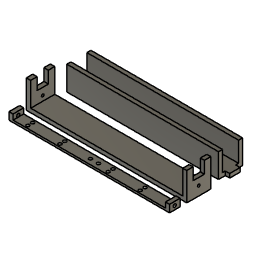
sampApp 20 v19 (Autodesk Fusion 360 design; units mm, degrees)
Autodesk Fusion 360 part; units mm, degrees
note: some values were not read from the file. Chosen so that the rebuilt part matches the saved one: which face or edge a step refers to.
sketch "Sketch1" plane through (0, 0, 0) normal (0, 0, 1) x (1, 0, 0)
  line L0 (0, 0) -> (70, 0)
  line L1 (70, 0) -> (70, 50)
  line L2 (70, 50) -> (0, 50)
  line L3 (0, 50) -> (0, 0)
  constraint horizontal L0
  constraint vertical L1
  constraint horizontal L2
  constraint vertical L3
  constraint coincident L0.start L3.end
extrude "Extrude1" add sketch "Sketch1" along normal blind 5 makes body 1
sketch "Sketch2" plane through (0, 0, 5) normal (0, 0, 1) x (-1, 0, 0)
  line L0 (0, -50) -> (0, 0)
  line L1 (0, 0) -> (-70, 0)
  line L2 (-70, 0) -> (-70, -50)
  line L3 (-70, -50) -> (0, -50)
  line L4 (-65, 0) -> (-70, 0)
  line L5 (-70, 0) -> (-70, -50)
  line L6 (-70, -50) -> (-65, -50)
  line L7 (-65, -50) -> (-65, 0)
  line L8 (0, 0) -> (-5, 0)
  line L9 (-5, 0) -> (-5, -50)
  line L10 (-5, -50) -> (0, -50)
  line L11 (0, -50) -> (0, 0)
  constraint horizontal L4
  constraint vertical L5
  constraint horizontal L6
  constraint vertical L7
  constraint coincident L2.end L3.start
  constraint coincident L1 L4.start
  constraint horizontal L8
  constraint vertical L9
  constraint horizontal L10
  constraint vertical L11
  constraint coincident L3 L9.end
  constraint coincident L0.end L1.start
extrude "Extrude2" add sketch "Sketch2" along normal blind 30 contours L0 L1 L3 L8 L9 L10 L11 | L1 L2 L3 L4 L5 L6 L7 bodies 1
extrude "Extrude3" cut 1 faces at (45, 50, 1.6667) along direction (0, -1, 0) blind 10 on bodies 1 bodies 1
sketch "Sketch3" plane through (0, 0, 0) normal (0, 0, 1) x (1, 0, 0)
  line L0 (5, 45) -> (65, 45)
  line L1 (65, 45) -> (65, 85)
  line L2 (65, 85) -> (5, 85)
  line L3 (5, 85) -> (5, 45)
  constraint horizontal L0
  constraint vertical L1
  constraint horizontal L2
  constraint vertical L3
extrude "Extrude4" add sketch "Sketch3" along normal blind 5 separate body makes body 2
sketch "Sketch4" plane through (0, 0, 5) normal (0, 0, 1) x (-1, 0, 0)
  line L0 (-5, -85) -> (-5, -45)
  line L1 (-5, -45) -> (-65, -45)
  line L2 (-65, -45) -> (-65, -85)
  line L3 (-65, -85) -> (-5, -85)
  line L4 (-65, -45) -> (-5, -45)
  line L5 (-5, -45) -> (-5, -50)
  line L6 (-5, -50) -> (-65, -50)
  line L7 (-65, -50) -> (-65, -45)
  line L8 (-5, -80) -> (-65, -80)
  line L9 (-65, -80) -> (-65, -85)
  line L10 (-65, -85) -> (-5, -85)
  line L11 (-5, -85) -> (-5, -80)
  constraint horizontal L4
  constraint vertical L5
  constraint horizontal L6
  constraint vertical L7
  constraint coincident L0 L5.end
  constraint coincident L1.end L2.start
  constraint horizontal L8
  constraint vertical L9
  constraint horizontal L10
  constraint vertical L11
  constraint coincident L2.end L3.start
  constraint coincident L0 L8.start
extrude "Extrude5" add sketch "Sketch4" along normal blind 25 contours L0 L2 L3 L8 L9 L10 L11 | L0 L1 L2 L4 L5 L6 L7 bodies 2
extrude "Extrude6" cut 1 faces at (5, 70, 1.6667) along direction (1, 0, 0) blind 0.5 on bodies 2 bodies 2
extrude "Extrude7" cut 1 faces at (65, 60, 1.6667) along direction (-1, 0, 0) blind 0.5 on bodies 2 bodies 2
sketch "Sketch5" plane through (0, 0, 35) normal (0, 0, 1) x (-1, 0, 0)
  line L0 (-5, -40) -> (0, -40)
  line L1 (0, -40) -> (0, 0)
  line L2 (0, 0) -> (-5, 0)
  line L3 (-5, 0) -> (-5, -40)
  line L4 (0, -15) -> (-5, -15)
  line L5 (-5, -15) -> (-5, -25)
  line L6 (-5, -25) -> (0, -25)
  line L7 (0, -25) -> (0, -15)
  line L8 (-70, -15) -> (-65, -15)
  line L9 (-65, -15) -> (-65, -25)
  line L10 (-65, -25) -> (-70, -25)
  line L11 (-70, -25) -> (-70, -15)
  constraint horizontal L4
  constraint vertical L5
  constraint horizontal L6
  constraint vertical L7
  constraint coincident L3 L5.end
  constraint coincident L1 L4.start
  constraint horizontal L8
  constraint vertical L9
  constraint horizontal L10
  constraint vertical L11
extrude "Extrude8" cut sketch "Sketch5" against normal blind 10 contours L8 L9 L10 L11 bodies 1
sketch "Sketch6" plane through (0, 0, 35) normal (0, 0, 1) x (-1, 0, 0)
  line L0 (-5, -40) -> (0, -40)
  line L1 (0, -40) -> (0, 0)
  line L2 (0, 0) -> (-5, 0)
  line L3 (-5, 0) -> (-5, -40)
  line L4 (0, -15) -> (-5, -15)
  line L5 (-5, -15) -> (-5, -25)
  line L6 (-5, -25) -> (0, -25)
  line L7 (0, -25) -> (0, -15)
  constraint horizontal L4
  constraint vertical L5
  constraint horizontal L6
  constraint vertical L7
  constraint coincident L3 L5.end
  constraint coincident L1 L4.start
extrude "Extrude9" cut sketch "Sketch6" against normal blind 10 contours L1 L3 L4 L5 L6 L7 bodies 1
sketch "Sketch7" plane through (0, 0, 5) normal (0, 0, 1) x (-1, 0, 0)
  line L0 (-65, -40) -> (-5, -40)
  line L1 (-5, -40) -> (-5, 0)
  line L2 (-5, 0) -> (-65, 0)
  line L3 (-65, 0) -> (-65, -40)
  line L4 (0, 15) -> (-70, 15)
  line L5 (-70, 15) -> (-70, 25)
  line L6 (-70, 25) -> (0, 25)
  line L7 (0, 25) -> (0, 15)
  constraint horizontal L4
  constraint vertical L5
  constraint horizontal L6
  constraint vertical L7
extrude "Extrude10" add sketch "Sketch7" along normal blind 5 separate body contours L4 L5 L6 L7 makes body 3
sketch "Sketch8" plane through (64.5, 0, 0) normal (1, 0, 0) x (0, 1, 0)
  line L0 (45, 0) -> (85, 0)
  line L1 (85, 0) -> (85, 30)
  line L2 (85, 30) -> (80, 30)
  line L3 (80, 30) -> (80, 5)
  line L4 (80, 5) -> (50, 5)
  line L5 (50, 5) -> (50, 30)
  line L6 (50, 30) -> (45, 30)
  line L7 (45, 30) -> (45, 0)
  line L8 (70, 5) -> (60, 5)
  line L9 (60, 5) -> (60, 0)
  line L10 (60, 0) -> (70, 0)
  line L11 (70, 0) -> (70, 5)
  constraint horizontal L8
  constraint vertical L9
  constraint horizontal L10
  constraint vertical L11
  constraint coincident L0 L9.end
  constraint coincident L4 L8.start
extrude "Extrude11" add sketch "Sketch8" along normal blind 7.5 contours L0 L4 L8 L9 L10 L11 bodies 2
extrude "Extrude12" cut 1 faces at (72, 63.3333, 3.3333) along direction (-1, 0, 0) blind 2 on bodies 2 bodies 2
sketch "Sketch9" plane through (5.5, 0, 0) normal (-1, 0, 0) x (0, -1, 0)
  line L0 (-85, 0) -> (-45, 0)
  line L1 (-45, 0) -> (-45, 30)
  line L2 (-45, 30) -> (-50, 30)
  line L3 (-50, 30) -> (-50, 5)
  line L4 (-50, 5) -> (-80, 5)
  line L5 (-80, 5) -> (-80, 30)
  line L6 (-80, 30) -> (-85, 30)
  line L7 (-85, 30) -> (-85, 0)
  line L8 (-60.2501, 5) -> (-70, 5)
  line L9 (-70, 5) -> (-70, 0)
  line L10 (-70, 0) -> (-60.2501, 0)
  line L11 (-60.2501, 0) -> (-60.2501, 5)
  constraint horizontal L8
  constraint vertical L9
  constraint horizontal L10
  constraint vertical L11
  constraint coincident L0 L9.end
  constraint coincident L4 L8.start
extrude "Extrude13" add sketch "Sketch9" along normal blind 5.5 contours L0 L4 L8 L9 L10 L11 bodies 2
move_body "Move1" bodies 3 to x (1, 0, 0) y (0, 1, 0) z (0, 0, 1) at (0, 0, -5)
extrude "Extrude14" cut 2 faces at (68.3333, 18.3333, 25) (3.3333, 18.3333, 25) along direction (0, 0, -1) blind 5 on bodies 1 bodies 1
hole "Hole1" at (0, 20, 11.2237) direction (1, 0, 0) diameter 3.3 depth 83 tip angle 118 bodies 1
sketch "Sketch10" plane through (0, 0, 5) normal (0, 0, 1) x (-1, 0, 0)
  line L0 (0, 25) -> (-70, 25)
  line L1 (-70, 25) -> (-70, 15)
  line L2 (-70, 15) -> (0, 15)
  line L3 (0, 15) -> (0, 25)
  line L4 (0, 15) -> (-5, 15)
  line L5 (-5, 15) -> (-5, 25)
  line L6 (-5, 25) -> (0, 25)
  line L7 (0, 25) -> (0, 15)
  line L8 (-70, 15) -> (-65, 15)
  line L9 (-65, 15) -> (-65, 25)
  line L10 (-65, 25) -> (-70, 25)
  line L11 (-70, 25) -> (-70, 15)
  constraint horizontal L4
  constraint vertical L5
  constraint horizontal L6
  constraint vertical L7
  constraint coincident L0 L5.end
  constraint coincident L2.end L3.start
  constraint horizontal L8
  constraint vertical L9
  constraint horizontal L10
  constraint vertical L11
  constraint coincident L0 L9.end
  constraint coincident L1.end L2.start
extrude "Extrude15" add sketch "Sketch10" along normal blind 5 contours L0 L2 L3 L4 L5 L6 L7 | L0 L1 L2 L8 L9 L10 L11 bodies 3
move_body "Move2" bodies 3 to x (1, 0, 0) y (0, 1, 0) z (0, 0, 1) at (0, 10, 0)
extrude "Extrude16" add 1 faces at (70, -8.3333, 3.3333) along direction (1, 0, 0) blind 103 on bodies 3 bodies 3
extrude "Extrude17" add 1 faces at (70, 5, 18.3333) along direction (1, 0, 0) blind 130 on bodies 1 bodies 1
extrude "Extrude18" add 1 faces at (64.5, 83.3333, 11.6667) along direction (1, 0, 0) blind 130 on bodies 2 bodies 2
extrude "Extrude19" add 1 faces at (70, 63.3333, 3.3333) along direction (1, 0, 0) blind 130 on bodies 2 bodies 2
extrude "Extrude20" add 1 faces at (64.5, 46.6667, 11.6667) along direction (1, 0, 0) blind 130 on bodies 2 bodies 2
extrude "Extrude21" cut 1 faces at (65, 35, 20) along direction (1, 0, 0) blind 130 on bodies 1 bodies 1
extrude "Extrude22" add 1 faces at (173, -8.3333, 3.3333) along direction (1, 0, 0) blind 33 on bodies 3 bodies 3
extrude "Extrude23" cut 1 faces at (65, -8.3333, 6.6667) along direction (1, 0, 0) blind 130 on bodies 3 bodies 3
extrude "Extrude24" cut 1 faces at (206, -8.3333, 3.3333) along direction (-1, 0, 0) blind 6 on bodies 3 bodies 3
extrude "Extrude25" cut 1 faces at (131.6667, -8.3333, 5) along direction (0, 0, -1) blind 2.5 on bodies 3 bodies 3
extrude "Extrude26" add 1 faces at (5, 5, 20) along direction (1, 0, 0) blind 0.5 on bodies 1 bodies 1
extrude "Extrude27" cut 1 faces at (131.6667, -8.3333, 2.5) along direction (0, 0, -1) blind 0.5 on bodies 3 bodies 3
extrude "Extrude28" add 1 faces at (198.3333, -15, 4) along direction (0, -1, 0) blind 2 on bodies 3 bodies 3
extrude "Extrude29" add 1 faces at (198.3333, -17, 4) along direction (0, -1, 0) blind 2 on bodies 3 bodies 3
extrude "Extrude30" cut 2 faces at (3.6667, 25, 30) (196.6667, 25, 30) along direction (0, 1, 0) blind 2 on bodies 1 bodies 1
extrude "Extrude31" cut 2 faces at (196.6667, 15, 25) (1.8333, 15, 30) along direction (0, -1, 0) blind 2 on bodies 1 bodies 1
extrude "Extrude32" add 2 faces at (3.6667, 70, 3.3333) (196.3333, 70, 1.6667) along direction (0, 1, 0) blind 2 on bodies 2 bodies 2
extrude "Extrude33" add 1 faces at (196.3333, 60, 3.3333) along direction (0, -1, 0) blind 2 on bodies 2 bodies 2
extrude "Extrude34" add 1 faces at (3.6667, 60.2501, 1.6667) along direction (0, -1, 0) blind 2 on bodies 2 bodies 2
extrude "Extrude35" cut 1 faces at (1.8333, 0, 13.3333) along direction (0, 1, 0) blind 5 on bodies 1 bodies 1
extrude "Extrude36" cut 1 faces at (1.8333, 40, 13.3333) along direction (0, -1, 0) blind 5 on bodies 1 bodies 1
extrude "Extrude37" add 1 faces at (131.5, 50, 21.6667) along direction (0, 1, 0) blind 5 on bodies 2 bodies 2
extrude "Extrude38" add 1 faces at (68.5, 80, 13.3333) along direction (0, -1, 0) blind 5 on bodies 2 bodies 2
extrude "Extrude39" cut 1 faces at (131.5, 85, 10) along direction (0, -1, 0) blind 5 on bodies 2 bodies 2
extrude "Extrude40" cut 1 faces at (68.5, 45, 10) along direction (0, 1, 0) blind 5 on bodies 2 bodies 2
extrude "Extrude41" cut 2 faces at (1.6667, -9.6667, 10) (196.6667, -9.6667, 10) along direction (0, 0, -1) blind 0.75 on bodies 3 bodies 3
sketch "Sketch11" plane through (0, 0, 2) normal (0, 0, 1) x (-1, 0, 0)
  line L0 (-195, 5) -> (-5, 5)
  line L1 (-5, 5) -> (-5, 19)
  line L2 (-5, 19) -> (-195, 19)
  line L3 (-195, 19) -> (-195, 5)
move_body "Move3" bodies 3 to x (1, 0, 0) y (0, 1, 0) z (0, 0, 1) at (0, 2, 0)
sketch "Sketch12" plane through (0, 0, 5) normal (0, 0, 1) x (-1, 0, 0)
  line L0 (-195, -35) -> (-5.5, -35)
  line L1 (-5.5, -35) -> (-5.5, -5)
  line L2 (-5.5, -5) -> (-195, -5)
  line L3 (-195, -5) -> (-195, -35)
sketch "Sketch13" plane through (0, 0, 2) normal (0, 0, 1) x (-1, 0, 0)
  line L0 (-195, 3) -> (-5, 3)
  line L1 (-5, 3) -> (-5, 17)
  line L2 (-5, 17) -> (-195, 17)
  line L3 (-195, 17) -> (-195, 3)
  circle A0 centre (-125, 7) radius 1
  circle A1 centre (-125, 13) radius 1
  circle A2 centre (-165, 13) radius 1
  circle A3 centre (-165, 7) radius 1
  circle A4 centre (-70, 7) radius 1
  circle A5 centre (-70, 13) radius 1
  circle A6 centre (-30, 7) radius 1
  circle A7 centre (-30, 13) radius 1
sketch "Sketch15" plane through (0, 0, 2) normal (0, 0, 1) x (-1, 0, 0)
  line L0 (-195, 3) -> (-5, 3)
  line L1 (-5, 3) -> (-5, 17)
  line L2 (-5, 17) -> (-195, 17)
  line L3 (-195, 17) -> (-195, 3)
  circle A0 centre (-95, 10) radius 1
  circle A1 centre (-105, 10) radius 1
  dimension "d97" = 2
  dimension "d98" = 2
  measures "d97" diameter of A0
  measures "d98" diameter of A1
hole "Hole6" at (0, -10, 4.625) direction (1, 0, 0) diameter 4 depth 225 tip angle 118 bodies 3
extrude "Extrude42" add 1 faces at (131.6667, -12.3333, 2) along direction (0, 0, 1) blind 0.625 on bodies 3 bodies 3
extrude "Extrude43" cut 1 faces at (196.3333, 58, 3.3333) along direction (0, 1, 0) blind 0.25 on bodies 2 bodies 2
extrude "Extrude44" cut 1 faces at (196.3333, 72, 1.6667) along direction (0, -1, 0) blind 0.25 on bodies 2 bodies 2
extrude "Extrude45" cut 1 faces at (3.6667, 72, 3.3333) along direction (0, -1, 0) blind 0.25 on bodies 2 bodies 2
extrude "Extrude46" cut 1 faces at (1.6667, -3, 3.9583) along direction (0, -1, 0) blind 0.25 on bodies 3 bodies 3
extrude "Extrude47" cut 1 faces at (1.6667, -17, 3.9583) along direction (0, 1, 0) blind 0.25 on bodies 3 bodies 3
sketch "Sketch16" plane through (0, 0, 2.625) normal (0, 0, 1) x (-1, 0, 0)
  line L0 (-5, 16.75) -> (-195, 16.75)
  line L1 (-195, 16.75) -> (-195, 10)
  line L2 (-195, 10) -> (-195, 3.25)
  line L3 (-195, 3.25) -> (-5, 3.25)
  line L4 (-5, 3.25) -> (-5, 10)
  line L5 (-5, 10) -> (-5, 16.75)
  circle A0 centre (-160, 7) radius 2
  circle A1 centre (-160, 13) radius 2
  circle A2 centre (-120, 7) radius 2
  circle A3 centre (-120, 13) radius 2
  circle A4 centre (-105, 10) radius 2
  circle A5 centre (-95, 10) radius 2
  circle A6 centre (-60, 7) radius 2
  circle A7 centre (-60, 13) radius 2
  circle A8 centre (-20, 7) radius 2
  circle A9 centre (-20, 13) radius 2
  dimension "d117" = 4
  dimension "d118" = 4
  dimension "d119" = 4
  dimension "d120" = 4
  dimension "d121" = 4
  dimension "d122" = 4
  dimension "d123" = 4
  measures "d117" diameter of A0
  measures "d118" diameter of A1
  measures "d119" diameter of A2
  measures "d120" diameter of A3
  measures "d121" diameter of A4
  measures "d122" diameter of A5
  measures "d123" diameter of A6
hole "Hole7" at (160, -7, 2.625) at (160, -13, 2.625) at (120, -7, 2.625) at (120, -13, 2.625) at (105, -10, 2.625) at (95, -10, 2.625) at (60, -7, 2.625) at (60, -13, 2.625) at (20, -7, 2.625) at (20, -13, 2.625) direction (0, 0, -1) diameter 4 depth 21 tip angle 118 bodies 3
extrude "Extrude48" cut 1 faces at (1.6667, -16.75, 3.9583) along direction (0, 1, 0) blind 0.25 on bodies 3 bodies 3
extrude "Extrude49" cut 1 faces at (196.3333, 58.25, 3.3333) along direction (0, 1, 0) blind 0.25 on bodies 2 bodies 2
extrude "Extrude50" cut 1 faces at (196.3333, 71.75, 1.6667) along direction (0, -1, 0) blind 0.25 on bodies 2 bodies 2
extrude "Extrude51" cut 1 faces at (3.6667, 71.75, 3.3333) along direction (0, -1, 0) blind 0.25 on bodies 2 bodies 2
extrude "Extrude52" cut 1 faces at (3.6667, 58.2501, 1.6667) along direction (0, 1, 0) blind 0.25 on bodies 2 bodies 2
sketch "Sketch14" plane through (0, 0, 2) normal (0, 0, 1) x (-1, 0, 0)
  circle A0 centre (-70, 13) radius 1
  circle A1 centre (-125, 13) radius 1
  circle A2 centre (-165, 7) radius 1
  circle A3 centre (-165, 13) radius 1
  circle A4 centre (-125, 7) radius 1
  circle A5 centre (-70, 7) radius 1
  circle A6 centre (-30, 13) radius 1
  circle A7 centre (-29.9996, 7.0002) radius 1
  line L0 (-195, 3) -> (-5, 3)
  line L1 (-5, 3) -> (-5, 17)
  line L2 (-5, 17) -> (-195, 17)
  line L3 (-195, 17) -> (-195, 3)
  circle A8 centre (-100, 7) radius 1
  circle A9 centre (-100, 13) radius 1
hole "Hole4" [suppressed]
